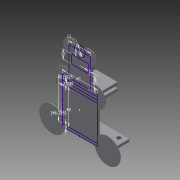
# Autodesk Inventor part: ToolHolderNeg
Saved by Autodesk Inventor 2014 SP1 (Build 180222100, 222)
## iProperties
Created: 2014-07-12
Part Number: ToolHolderNeg
Material: Generic
Document SubType Name: Modeling
Designer: Erin
Density: 1 g/cm^3
Appearance: Default
Author: Erin
Autodesk Inventor part; units mm, degrees
ref_plane "YZ Plane" through (0, 0, 0) normal (1, 0, 0) x (0, 1, 0)
ref_plane "XZ Plane" through (0, 0, 0) normal (0, 1, 0) x (-1, 0, 0)
ref_plane "XY Plane" through (0, 0, 0) normal (0, 0, 1) x (1, 0, 0)
sketch "Sketch1" plane through (0, 0, 0) normal (0, 1, 0) x (-1, 0, 0)
  line L0 (-20, 26.075) -> (20, 26.075)
  line L1 (20, 26.075) -> (20, -26.075)
  line L2 (20, -26.075) -> (-20, -26.075)
  line L3 (-20, -26.075) -> (-20, 26.075)
  line L4 (-20, 23.15) -> (20, 23.15)
  line L5 (-20, 19.85) -> (20, 19.85)
  line L6 (-20, 16.925) -> (20, 16.925)
  line L7 (-20, -23.075) -> (20, -23.075)
  line L8 (-12.5, 26.075) -> (12.5, 26.075)
  line L9 (12.5, 26.075) -> (12.5, 59.075)
  line L10 (12.5, 59.075) -> (-12.5, 59.075)
  line L11 (-12.5, 59.075) -> (-12.5, 26.075)
  line L12 (-9.5, 51.075) -> (9.5, 51.075)
  line L13 (9.5, 51.075) -> (9.5, 41.075)
  line L14 (9.5, 41.075) -> (-9.5, 41.075)
  line L15 (-9.5, 41.075) -> (-9.5, 51.075)
  circle A0 centre (0, 59.075) radius 6
  point P0 (0, 0)
  point P1 (0, -26.075)
  point P2 (20, 0)
  point P3 (0, 26.075)
  point P4 (0, 51.075)
  dimension "d0" = 2.925
  dimension "d1" = 3.3
  dimension "d2" = 2.925
  dimension "d3" = 3
  dimension "d4" = 40
  dimension "d17" = 40
  dimension "d18" = 46.225
  dimension "d27" = 25
  dimension "d28" = 3
  dimension "d29" = 15
  dimension "d30" = 10
  dimension "d31" = 8
  dimension "d32" = 12
  constraints: 32 end point, 9 point on line, 7 perpendicular, 6 parallel, 5 midpoint, 3 horizontal, 3 vertical alignment, 1 centre point, 1 coincident, 1 horizontal alignment
  measures "d0" distance between parallel lines of L4 L0
  measures "d1" distance between parallel lines of L5 L4
  measures "d2" distance between parallel lines of L6 L5
  measures "d3" distance between parallel lines of L7 L2
  measures "d4" distance between parallel lines of L7 L6
  measures "d17" distance of L0.start L0.end
  measures "d18" distance between parallel lines of L7 L4
  measures "d27" distance of L9.end L10.end
  measures "d28" distance between parallel lines of L15 L11
  measures "d29" distance between parallel lines of L14 L0
  measures "d30" distance of L12.end L13.end
  measures "d31" distance between parallel lines of L10 L12
  measures "d32" diameter of A0
extrude "Extrusion1" add sketch "Sketch1" along normal blind 3 contours L0 L1 L4 L3 | L4 L1 L5 L3 | L5 L1 L6 L3 | L6 L1 L7 L3 | L7 L1 L2 L3
extrude "Extrusion2" add sketch "Sketch1" along normal blind 23.5 contours L0 L1 L4 L3 | L5 L1 L6 L3
extrude "Extrusion3" add sketch "Sketch1" along normal blind 23 contours L7 L1 L2 L3
sketch "Sketch2" plane through (0, 23.5, 0) normal (0, 1, 0) x (1, 0, 0)
  line L0 (20, -23.15) -> (-20, -23.15) projected
  line L1 (-20, -26.075) -> (20, -26.075) projected
  circle A0 centre (-10, -23.15) radius 2.075
  line L2 (0, 35.4455) -> (0, -34.4872) construction
  circle A1 centre (10, -23.15) radius 2.075
  point P0 (0, 0)
  dimension "d11" = 4.15
  dimension "d12" = 10
  dimension "d13" = 4.15
  dimension "d14" = 10
  constraints: 2 centre point, 2 end point, 2 point on line, 1 perpendicular, 1 vertical
  measures "d11" diameter of A0
  measures "d12" distance from line of A0.centre L2
  measures "d13" diameter of A1
  measures "d14" distance from line of A1.centre L2
extrude "Extrusion4" cut sketch "Sketch2" against normal blind 20.5
sketch "Sketch3" plane through (20, 0, -26.075) normal (0, 0, -1) x (-1, 0, 0)
  line L0 (0, 23) -> (-14, 23)
  line L1 (-14, 23) -> (-14, 0)
  line L2 (-14, 0) -> (0, 0)
  line L3 (0, 0) -> (0, 23)
  circle A0 centre (-7, 18) radius 2.25
  circle A1 centre (-7, 5) radius 2.25
  point P0 (20, 0)
  point P1 (-7, 23)
  dimension "d19" = 4.5
  dimension "d20" = 7
  dimension "d21" = 5
  dimension "d22" = 4.5
  dimension "d23" = 7
  dimension "d24" = 5
  constraints: 8 end point, 2 centre point, 2 parallel, 1 horizontal, 1 midpoint, 1 perpendicular, 1 vertical alignment
  measures "d19" diameter of A0
  measures "d20" distance from line of A0.centre L1
  measures "d21" distance from line of A0.centre L0
  measures "d22" diameter of A1
  measures "d23" distance from line of A1.centre L1
  measures "d24" distance from line of A1.centre L2
extrude "Extrusion5" add sketch "Sketch3" against normal blind 3
mirror "Mirror1" about plane through (0, 0, 0) normal (1, 0, 0) of "Extrusion5"
extrude "Extrusion6" add sketch "Sketch1" along normal blind 3 contours L11 L10 A0 L9 L0 | L10 A0 | L12 L13 L14 L15 picked at (-1.1361, 55.5701)
extrude "Extrusion7" cut sketch "Sketch1" along normal blind 3 contours A0 L10 | L10 A0
extrude "Extrusion8" add sketch "Sketch1" along normal blind 10 contours L12 L13 L14 L15
fillet "Fillet1" radius 4 2 edges at (0, 3, 51.075) (0, 10, 51.075)
fillet "Fillet2" radius 5 3 edges at (0, 3, 26.075) (12.5, 1.5, 26.075) (-12.5, 1.5, 26.075)
sketch "Sketch4" plane through (0, 0, 0) normal (0, -1, 0) x (1, 0, 0)
  circle A0 centre (31.8052, -24.575) radius 14.5819
  circle A1 centre (17.2233, 21.9719) radius 12.1989
  circle A2 centre (10.6017, 57.311) radius 8.6187
  point P0 (0, 0)
  constraints: 3 centre point
extrude "Extrusion9" add sketch "Sketch4" against normal blind 0.6
mirror "Mirror2" about plane through (0, 0, 0) normal (1, 0, 0) of "Extrusion9"
equation "\"sp\" = 0.15"
body "Solid1"
